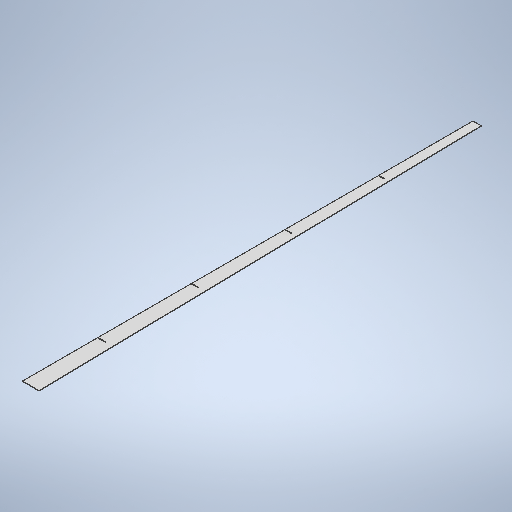
# Autodesk Inventor part: BSH 022 rib 2
Saved by Autodesk Inventor 2025 (Build 290162010, 162A)
## iProperties
Created: 2024-07-23
Part Number: BSH 022 rib 2
Material: Stainless Steel
Document SubType Name: Sheet Metal
Designer: admin
Density: 8 g/cm^3
Sheet Metal Rule: AISI304 3mm Die 32
Appearance: Default
Author: admin
Autodesk Inventor part; units mm, degrees
ref_plane "YZ Plane" through (0, 0, 0) normal (1, 0, 0) x (0, 1, 0)
ref_plane "XZ Plane" through (0, 0, 0) normal (0, 1, 0) x (-1, 0, 0)
ref_plane "XY Plane" through (0, 0, 0) normal (0, 0, 1) x (1, 0, 0)
sketch "Sketch1" plane through (0, 0, 0) normal (0, 0, 1) x (1, 0, 0)
  line L0 (1200, 2950) -> (-1200, 2950)
  line L1 (-1200, 2950) -> (-1200, 0)
  line L2 (-1200, 0) -> (1200, 0)
  line L3 (1200, 0) -> (1200, 2950)
  line L4 (1150, 2950) -> (1150, 0)
  line L5 (-1150, 0) -> (-1150, 2950) construction
  line L6 (0, 2950) -> (0, 50) construction
  line L7 (-1100, 200) -> (-950, 50)
  line L8 (-1200, 100) -> (-1100, 100)
  line L9 (-1100, 100) -> (-1100, 0)
  line L10 (-1100, 200) -> (-1150, 2950)
  arc A0 (-1100.4545, 224.9959) -> (-1082.3223, 182.3223) centre (-1100, 200) ccw
  arc A1 (-1082.3223, 182.3223) -> (-1100.4545, 224.9959) centre (-1100, 200) ccw construction
  line L11 (-1200, 255) -> (-1101, 255)
  line L12 (0, 50) -> (-950, 50)
  line L13 (0, 50) -> (0, 0)
  line L14 (1505.3449, -225.894) -> (355.3449, -225.894)
  dimension "d3" = 2400
  dimension "d4" = 2950
  dimension "d5" = 50
  dimension "d6" = 100
  dimension "d7" = 50
  dimension "d8" = 2695
  dimension "d9" = 135
  dimension "d10" = 950
  dimension "d11" = 1150
  dimension "d12" = 136.042
  dimension "d13" = 50
  dimension "d14" = 100
  dimension "d15" = 212.132
  dimension "d17" = 55
  dimension "d20" = 200
  measures "d3" distance of L3.start L1.end
  measures "d4" distance of L1.end L1.start
  measures "d5" diameter of A0
  measures "d6" distance of L8.start L8.end
  measures "d7" distance between parallel lines of L1 L5
  measures "d8" distance between parallel lines of L0 L11
  measures "d9" angle of L12 L7
  measures "d10" distance of L6.end L7.end
  measures "d11" distance of L14.start L14.end
  measures "d12" angle of L7 L10
  measures "d13" distance between parallel lines of L2 L12
  measures "d14" distance from line of L1 L10.start
  measures "d15" distance of L10.start L7.end
  measures "d17" vertical distance of L10.start L11.end
  measures "d20" distance from line of L2 A1.centre
extrude "Plate1" add sketch "Sketch1" along normal blind 3 contours L10 L11 L1 L0
sketch "Sketch2" plane through (0, 0, 3) normal (0, 0, 1) x (1, 0, 0)
  line L0 (-1101, 255) -> (-1200, 255) projected
  line L1 (-1150, 2950) -> (-1101, 255) projected
  line L2 (-1200, 2950) -> (-1150, 2950) projected
  line L3 (-1200, 255) -> (-1200, 2950) projected
  line L4 (-1101, 255) -> (-1150, 2950) projected
  line L5 (-1158.7453, 1267.3175) -> (-1158.6871, 1264.1181)
  line L6 (-1158.6871, 1264.1181) -> (-1119.3606, 1264.8331) construction
  line L7 (-1150, 2950) -> (-1101, 255) projected
  line L8 (-1158.6871, 1264.1181) -> (-1200, 1263.3669)
  line L9 (-1158.7453, 1267.3175) -> (-1200, 1266.5675)
  line L10 (-1200, 703.2744) -> (-1153.5904, 704.1182)
  line L11 (-1153.5904, 704.1182) -> (-1153.6486, 707.3177)
  line L12 (-1153.5904, 704.1182) -> (-1109.1805, 704.9256) construction
  line L13 (-1153.6486, 707.3177) -> (-1200, 706.4749)
  line L14 (-1200, 1823.4595) -> (-1163.7705, 1824.1182)
  line L15 (-1163.7705, 1824.1182) -> (-1163.8287, 1827.3177)
  line L16 (-1163.8287, 1827.3177) -> (-1200, 1826.66)
  line L17 (-1163.7705, 1824.1182) -> (-1129.5407, 1824.7406) construction
  line L18 (-1200, 2383.552) -> (-1168.8606, 2384.1182)
  line L19 (-1168.8606, 2384.1182) -> (-1168.9188, 2387.3177)
  line L20 (-1168.8606, 2384.1182) -> (-1139.7209, 2384.648) construction
  line L21 (-1168.9188, 2387.3177) -> (-1200, 2386.7526)
  point P0 (0, 0)
  point P1 (-1119.3606, 1264.8331)
  dimension "d32" = 450
  dimension "d34" = 46.4173
  dimension "d36" = 41.3197
  dimension "d39" = 36.2355
  dimension "d42" = 31.1445
  dimension "d43" = 560
  dimension "d44" = 3.2
  dimension "d45" = 560
  dimension "d46" = 3.2
  dimension "d47" = 560
  dimension "d48" = 3.2
  dimension "d49" = 3.2
  constraints: 32 end point, 11 perpendicular, 6 parallel, 4 point on line, 1 collinear, 9 other
  measures "d32" distance from line of L10 L0.start
  measures "d34" distance of L10.start L10.end
  measures "d36" distance of L8.end L5.end
  measures "d39" distance of L14.start L14.end
  measures "d42" distance of L18.end L18.start
  measures "d43" distance of L6.end L12.end
  measures "d44" distance between parallel lines of L10 L13
  measures "d45" distance of L17.end L6.end
  measures "d46" distance between parallel lines of L8 L9
  measures "d47" distance of L20.end L17.end
  measures "d48" distance between parallel lines of L14 L16
  measures "d49" distance between parallel lines of L18 L21
extrude "Extrusion1" cut sketch "Sketch2" against normal through all contours L3 L13 L11 L10 | L21 L19 L18 L3 | L3 L9 L5 L8 | L16 L15 L14 L3
equation "\"d11\" = d10 + d18"
equation "\"d14\" = d6"
equation "\"d32\" = Stringer1_hight"
equation "\"d43\" = Stringer1_step"
equation "\"d45\" = Stringer1_step"
equation "\"d47\" = Stringer1_step"
equation "\"d2\" = Thickness"
equation "\"BendReliefWidth\" = Thickness"
equation "\"BendReliefDepth\" = 0.5 * Thickness"
equation "\"CornerReliefSize\" = 4 * Thickness"
equation "\"MinimumRemnant\" = 2 * Thickness"
equation "\"TransitionRadius\" = BendRadius"
equation "\"JacobiRadiusSize\" = BendRadius"
equation "\"GapSize\" = Thickness"
equation "\"d18\" = d19"
equation "\"Stringer1_hight\" = 450"
equation "\"Stringer1_step\" = 560"
equation "\"Thickness\" = 3"
equation "\"BendRadius\" = 5"
equation "\"d19\" = 200"
body "Solid1"
